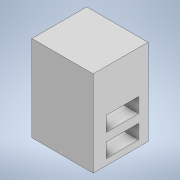
# Autodesk Inventor part: Part4
Saved by Autodesk Inventor 2021 (Build 250183000, 183)
## iProperties
Created: 2021-02-28
Part Number: Part4
Material: Generic
Document SubType Name: Modeling
Designer: K.V
Density: 1 g/cm^3
Appearance: Default
Author: K.V
Autodesk Inventor part; units mm, degrees
ref_plane "YZ Plane" through (0, 0, 0) normal (1, 0, 0) x (0, 1, 0)
ref_plane "XZ Plane" through (0, 0, 0) normal (0, 1, 0) x (-1, 0, 0)
ref_plane "XY Plane" through (0, 0, 0) normal (0, 0, 1) x (1, 0, 0)
sketch "Sketch1" plane through (0, 0, 0) normal (1, 0, 0) x (0, 1, 0)
  line L0 (10.812, 12.057) -> (-14.132, 12.057)
  line L1 (-14.132, 12.057) -> (-14.132, -3.8443)
  line L2 (-14.132, -3.8443) -> (10.812, -3.8443)
  line L3 (10.812, -3.8443) -> (10.812, 12.057)
  point P0 (0, 0)
  constraints: 8 end point, 2 parallel, 1 horizontal, 1 perpendicular
extrude "Extrusion1" add sketch "Sketch1" along normal blind 17.78
sketch "Sketch2" plane through (17.78, 0, 0) normal (1, 0, 0) x (0, 0, -1)
  line L0 (-8.2866, -8.1756) -> (1.1098, -8.1756)
  line L1 (1.1098, -8.1756) -> (1.1098, -12.3189)
  line L2 (1.1098, -12.3189) -> (-8.2866, -12.3189)
  line L3 (-8.2866, -12.3189) -> (-8.2866, -8.1756)
  line L4 (-8.2866, -1.4428) -> (1.1098, -1.4428)
  line L5 (1.1098, -1.4428) -> (1.1098, -5.734)
  line L6 (1.1098, -5.734) -> (-8.2866, -5.734)
  line L7 (-8.2866, -5.734) -> (-8.2866, -1.4428)
  point P0 (0, 0)
  constraints: 16 end point, 4 parallel, 2 horizontal, 2 perpendicular, 2 point on line
extrude "Extrusion2" cut sketch "Sketch2" against normal blind 10.16
sketch "Sketch3" plane through (0, 0, 0) normal (-1, 0, 0) x (0, 0, 1)
  line L0 (8.2866, -12.3189) -> (8.2866, -8.1756) projected
  line L1 (0.5236, -9.8392) -> (8.2866, -9.8392)
  line L2 (8.2866, -9.8392) -> (8.2866, -11.7154)
  line L3 (8.2866, -11.7154) -> (0.5236, -11.7154)
  line L4 (0.5236, -11.7154) -> (0.5236, -9.8392)
  point P0 (0, 0)
  constraints: 8 end point, 2 parallel, 1 horizontal, 1 perpendicular, 1 point on line
extrude "Extrusion3" cut sketch "Sketch3" against normal blind 25.4
body "Solid1"
